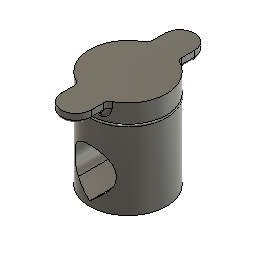
Cylinder Valve stopper v11 (Autodesk Fusion 360 design; units mm, degrees)
Autodesk Fusion 360 part; units mm, degrees
sketch "Sketch1" plane through (0, 0, 0) normal (0, 0, 1) x (1, 0, 0)
  line L0 (0, 0) -> (12.96, 0)
  line L1 (12.96, 0) -> (12.96, 30)
  line L2 (12.96, 30) -> (0, 30)
  line L3 (0, 30) -> (0, 0)
  arc A0 (12.96, 26.0571) -> (12.96, 26.7429) centre (12.89, 26.4) ccw
  dimension "d1" = 30
  dimension "d2" = 12.96
  dimension "d14" = 26.4
  dimension "d15" = 0.35
  dimension "d16" = 0.07
  constraint coincident L0.start L3.end
  constraint horizontal L0
  constraint perpendicular L0 L1
  constraint perpendicular L1 L2
  constraint perpendicular L0 L3
  constraint coincident L1 A0.start
  constraint coincident L1 A0.end
  measures "d1" distance of L0.end L1.end
  measures "d2" distance of L0.start L0.end
  measures "d14" distance of L0 A0.centre
  measures "d15" radius of A0
  measures "d16" distance of L1 A0.centre
revolve "Revolve1" add sketch "Sketch1" angle 360 about axis through (0, 30, 0) along (0, -1, 0)
sketch "Sketch2" plane through (0, 0, 0) normal (0, 0, 1) x (1, 0, 0)
  line L0 (0, 11.1) -> (0, 0) construction
  line L1 (-4.7291, 5.9391) -> (0, 1.6056)
  line L2 (4.7291, 5.9391) -> (0, 1.6056)
  arc A0 (4.7291, 5.9391) -> (-4.7291, 5.9391) centre (0, 11.1) ccw
  dimension "d4" = 11.1
  dimension "d5" = 14
  dimension "d8" = 95
  constraint coincident L0.start A0.centre
  constraint coincident L0.end origin
  constraint vertical L0
  constraint coincident L0 L1.end
  constraint equal L1 L2
  constraint tangent L2 A0
  measures "d4" distance of L0.end L0.start
  measures "d5" diameter of A0
  measures "d8" angle of L1 L2
extrude "Extrude1" cut sketch "Sketch2" along normal through all and the other way through all
sketch "Sketch3" plane through (0, 30, 0) normal (0, 1, 0) x (-1, 0, 0)
  circle A0 centre (0, 0) radius 12.96
sketch "Sketch4" plane through (0, 30, 0) normal (0, 1, 0) x (-1, 0, 0)
  line L0 (5, -17.5) -> (5, 17.5)
  arc A0 (5, 17.5) -> (-5, 17.5) centre (0, 17.5) ccw
  line L1 (-5, 17.5) -> (-5, -17.5)
  arc A1 (-5, -17.5) -> (5, -17.5) centre (0, -17.5) ccw
  circle A2 centre (0, 0) radius 12.96
  line L2 (0, 17.5) -> (0, -17.5) construction
  dimension "d9" = 35
  dimension "d13" = 10
  constraint vertical L0
  constraint tangent L0 A0
  constraint parallel L0 L1
  constraint tangent L1 A1
  constraint tangent L0 A1
  constraint tangent A0 L1
  constraint coincident A0.centre L2.start
  constraint coincident A1.centre L2.end
  constraint midpoint A2.centre L2
  measures "d9" distance of A0.centre A1.centre
  measures "d13" distance of L0 L1
extrude "Extrude2" add sketch "Sketch3" sketch "Sketch4" along normal blind 3 of sketch 2 contours L0 L1 A1 A2 | L0 A0 L1 A2
fillet "Fillet2" radius 1 6 edges at (5, 30, -14.7283) (0, 30, -22.5) (-5, 30, -14.7283) (-5, 30, 14.7283) (0, 30, 22.5) (5, 30, 14.7283)
fillet "Fillet3" radius 2 10 edges at (-5, 32, -11.9567) (-4.6987, 30.2846, -12.0782) (0, 30, -12.96) (4.6987, 30.2846, -12.0782) (5, 32, -11.9567) (5, 32, 11.9567) (4.6987, 30.2846, 12.0782) (0, 30, 12.96) (-4.6987, 30.2846, 12.0782) (-5, 32, 11.9567)
chamfer "Chamfer1" distance 0.1 angle 45 1 edges at (-12.083, 26.0571, -4.6865)
